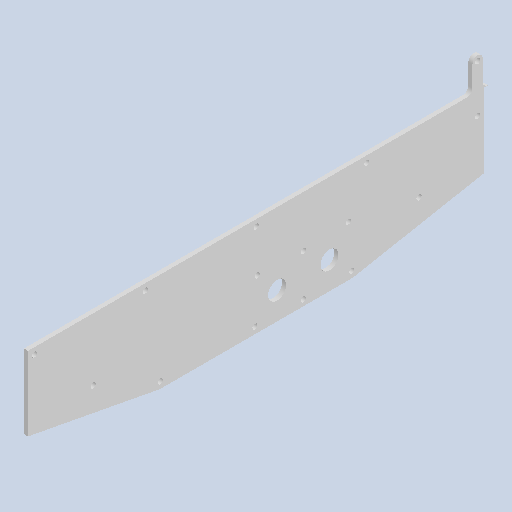
# Autodesk Inventor part: InsideChassiPlate3.0
Saved by Autodesk Inventor 2023 (Build 270158000, 158)
## iProperties
Created: 2022-09-18
Part Number: InsideChassiPlate3.0
Material: Generic
Document SubType Name: Modeling
Designer: deli
Density: 1 g/cm^3
Appearance: Default
Mass: 76.7316 g
Surface Area: 518.075 cm^2
Volume: 76.7316 cm^3
Author: deli
Autodesk Inventor part; units mm, degrees
ref_plane "YZ Plane" through (0, 0, 0) normal (1, 0, 0) x (0, 1, 0)
ref_plane "XZ Plane" through (0, 0, 0) normal (0, 1, 0) x (-1, 0, 0)
ref_plane "XY Plane" through (0, 0, 0) normal (0, 0, 1) x (1, 0, 0)
sketch "Sketch1" plane through (0, 0, 0) normal (1, 0, 0) x (0, 1, 0)
  line L0 (153.267, 41.7418) -> (153.267, -105.149) projected
  arc A0 (153.267, -105.149) -> (153.3544, -106.0799) centre (158.267, -105.149) ccw projected
  line L1 (153.3544, -106.0799) -> (172.4208, -206.7036) projected
  line L2 (172.4208, -206.7036) -> (577.767, -206.7036) projected
  line L3 (253.267, -105.2209) -> (253.267, 143.2964) projected
  line L4 (253.267, 143.2964) -> (172.4208, 143.2964) projected
  line L5 (172.4208, 143.2964) -> (153.3544, 42.6727) projected
  arc A1 (153.3544, 42.6727) -> (153.267, 41.7418) centre (158.267, 41.7418) ccw projected
  circle A2 centre (224.267, 53.2964) radius 2 projected
  circle A3 centre (224.267, -116.7036) radius 2 projected
  circle A4 centre (212.8897, -201.7036) radius 2 projected
  circle A5 centre (192.186, -102.5532) radius 2 projected
  circle A6 centre (158.267, -30.806) radius 2 projected
  circle A7 centre (157.883, -67.9775) radius 2 projected
  circle A8 centre (190.1509, -67.9775) radius 2 projected
  circle A9 centre (174.017, -88.0464) radius 7 projected
  circle A10 centre (174.017, -47.9087) radius 7 projected
  circle A11 centre (181.267, -156.7036) radius 2 projected
  circle A12 centre (181.267, 93.2964) radius 2 projected
  circle A13 centre (224.267, 138.2964) radius 2 projected
  circle A14 centre (191.4689, -32.5466) radius 2 projected
  circle A15 centre (224.267, -31.7036) radius 2 projected
  circle A16 centre (158.267, 41.7418) radius 2 projected
  circle A17 centre (158.267, -105.149) radius 2 projected
  circle A18 centre (249.267, -201.7036) radius 2 projected
  circle A19 centre (249.267, -201.7036) radius 2 projected
  line L6 (249.267, -197.7036) -> (233.267, -197.7036)
  line L7 (233.267, -205.7036) -> (249.267, -205.7036)
  line L8 (229.267, 143.2964) -> (229.267, -193.7036)
  line L9 (229.267, -209.7036) -> (229.267, -206.7036)
  arc A20 (249.267, -205.7036) -> (249.267, -197.7036) centre (249.267, -201.7036) ccw
  arc A21 (229.267, -193.7036) -> (233.267, -197.7036) centre (233.267, -193.7036) ccw
  arc A22 (233.267, -205.7036) -> (229.267, -209.7036) centre (233.267, -209.7036) ccw
  line L10 (577.767, -206.7036) -> (577.767, -186.7036) projected
  line L11 (577.767, -186.7036) -> (253.267, -105.2209) projected
  point P0 (0, 0)
  point P1 (229.267, -205.7036)
  point P2 (229.267, -197.7036)
  point P3 (253.267, -167.2852)
  point P4 (280.5019, -186.7036)
  point P5 (283.5543, -206.7036)
  point P6 (253.267, -175.0536)
  point P7 (253.267, -176.7309)
  point P8 (230.6212, -206.7036)
  point P9 (214.9796, -206.7036)
  point P10 (253.267, -165.3763)
  point P11 (253.267, -167.0536)
  dimension "d8" = 8
  dimension "d9" = 4
  dimension "d10" = 5
  dimension "d11" = 5
  constraints: 8 end point, 6 point on circle, 6 point on line, 5 tangent, 3 centre point, 2 equal radius, 2 vertical, 1 coincident, 1 horizontal, 1 parallel
  measures "d8" distance between parallel lines of L7 L6
  measures "d9" distance from line of L7 A18.centre
  measures "d10" distance from line of L8 A15.centre
  measures "d11" distance from line of L9 A3.centre
extrude "Extrusion1" add sketch "Sketch1" along normal blind 3.175 contours A1 L5 L4 L8 A21 L6 A20 L7 A22 L2 L1 A0 L0 | L2 A22 L9
equation "\"d9\" = 0.5 * d8"
equation "\"d11\" = d10"
body "Solid1"
